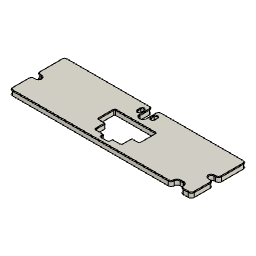
Frame Cover Plate (Autodesk Fusion 360 design; units mm, degrees)
Autodesk Fusion 360 part; units mm, degrees
sketch "Sketch1" plane through (0, 0, 0) normal (0, 0, 1) x (1, 0, 0) in component "Cover"
  line L0 (69.75, 5.3) -> (63.75, 5.3)
  line L1 (47.25, 23.3) -> (47.25, 12.3)
  line L2 (69.75, 12.3) -> (69.75, 5.3)
  line L3 (74.75, 12.3) -> (69.75, 12.3)
  line L4 (63.75, 5.3) -> (63.75, 2.8)
  line L5 (52.25, 12.3) -> (52.25, 5.3)
  line L6 (63.75, 2.8) -> (58.25, 2.8)
  line L7 (47.25, 23.3) -> (74.75, 23.3)
  line L8 (47.25, 12.3) -> (52.25, 12.3)
  line L9 (58.25, 2.8) -> (58.25, 5.3)
  line L10 (74.75, 23.3) -> (74.75, 12.3)
  line L11 (52.25, 5.3) -> (58.25, 5.3)
  circle A0 centre (12.7254, 3.937) radius 0.45 construction
  line L12 (11.8504, 5.602) -> (11.8504, 7.352) construction
  line L13 (13.6004, 5.602) -> (11.8504, 5.602) construction
  line L14 (27.5938, 3.7375) -> (27.5938, 5.5875) construction
  line L15 (29.4438, 3.7375) -> (27.5938, 3.7375) construction
  circle A1 centre (28.5188, 4.6625) radius 0.5 construction
  circle A2 centre (26.0188, 4.6625) radius 0.925 construction
  circle A3 centre (12.7254, 6.477) radius 0.45 construction
  circle A4 centre (72.7364, 31.0857) radius 1.225 construction
  circle A5 centre (77.7364, 31.0857) radius 1.225 construction
  circle A6 centre (10.1854, 6.477) radius 0.875 construction
  circle A7 centre (10.1854, 3.937) radius 0.875 construction
  circle A8 centre (43.897, 31.0857) radius 1.225 construction
  circle A9 centre (48.897, 31.0857) radius 0.7 construction
  circle A10 centre (10.1854, 3.937) radius 0.45 construction
  circle A11 centre (48.897, 31.0857) radius 1.225 construction
  circle A12 centre (10.1854, 6.477) radius 0.45 construction
  circle A13 centre (77.7364, 31.0857) radius 0.7 construction
  line L16 (11.8504, 7.352) -> (13.6004, 7.352) construction
  circle A14 centre (35.3679, 34.0015) radius 0.875 construction
  circle A15 centre (8.4979, 19.224) radius 0.925 construction
  line L17 (13.6004, 7.352) -> (13.6004, 5.602) construction
  line L18 (7.5729, 15.149) -> (9.4229, 15.149) construction
  line L19 (37.0329, 34.8765) -> (38.7829, 34.8765) construction
  line L20 (9.4229, 15.149) -> (9.4229, 13.299) construction
  line L21 (9.4229, 13.299) -> (7.5729, 13.299) construction
  circle A16 centre (35.3679, 31.4615) radius 0.45 construction
  line L22 (28.3943, 33.0249) -> (26.6443, 33.0249) construction
  circle A17 centre (37.9079, 34.0015) radius 0.45 construction
  line L23 (7.5729, 13.299) -> (7.5729, 15.149) construction
  circle A18 centre (8.4979, 16.724) radius 0.925 construction
  circle A19 centre (43.897, 31.0857) radius 0.7 construction
  circle A20 centre (23.5188, 4.6625) radius 0.5 construction
  circle A21 centre (12.7254, 3.937) radius 0.875 construction
  circle A22 centre (8.4979, 14.224) radius 0.5 construction
  circle A23 centre (72.7364, 31.0857) radius 0.7 construction
  circle A24 centre (23.5188, 4.6625) radius 0.925 construction
  line L24 (38.7829, 34.8765) -> (38.7829, 33.1265) construction
  circle A25 centre (35.3679, 34.0015) radius 0.45 construction
  line L25 (29.4438, 5.5875) -> (29.4438, 3.7375) construction
  circle A26 centre (26.0188, 4.6625) radius 0.5 construction
  line L26 (37.0329, 33.1265) -> (37.0329, 34.8765) construction
  circle A27 centre (27.5193, 31.3599) radius 0.45 construction
  line L27 (38.7829, 33.1265) -> (37.0329, 33.1265) construction
  circle A28 centre (8.4979, 19.224) radius 0.5 construction
  circle A29 centre (35.3679, 31.4615) radius 0.875 construction
  circle A30 centre (24.9793, 33.8999) radius 0.875 construction
  circle A31 centre (8.4979, 21.724) radius 0.925 construction
  line L28 (27.5938, 5.5875) -> (29.4438, 5.5875) construction
  arc A32 (83.6167, 10.5889) -> (84.2667, 10.5889) centre (83.9417, 10.5889) ccw construction
  arc A33 (83.3167, 10.6139) -> (84.5667, 10.6139) centre (83.9417, 10.6139) ccw construction
  arc A34 (79.9067, 6.3739) -> (78.6567, 6.3739) centre (79.2817, 6.3739) ccw construction
  circle A35 centre (8.4979, 16.724) radius 0.5 construction
  line L29 (26.6443, 33.0249) -> (26.6443, 34.7749) construction
  circle A36 centre (112.7141, 21.9272) radius 0.925 construction
  circle A37 centre (24.9793, 31.3599) radius 0.875 construction
  line L30 (113.6391, 13.5022) -> (111.7891, 13.5022) construction
  circle A38 centre (81.6116, 12.4939) radius 0.35 construction
  line L31 (78.6567, 6.3739) -> (78.6567, 5.8739) construction
  line L32 (43.1948, 5.6637) -> (45.0448, 5.6637) construction
  circle A39 centre (37.9079, 31.4615) radius 0.45 construction
  circle A40 centre (36.6198, 4.7387) radius 0.925 construction
  circle A41 centre (27.5193, 31.3599) radius 0.875 construction
  circle A42 centre (39.1198, 4.7387) radius 0.925 construction
  line L33 (26.6443, 34.7749) -> (28.3943, 34.7749) construction
  line L34 (28.3943, 34.7749) -> (28.3943, 33.0249) construction
  line L35 (45.0448, 3.8137) -> (43.1948, 3.8137) construction
  circle A43 centre (36.6198, 4.7387) radius 0.5 construction
  line L36 (111.7891, 15.3522) -> (113.6391, 15.3522) construction
  circle A44 centre (27.5193, 33.8999) radius 0.45 construction
  line L37 (111.7891, 13.5022) -> (111.7891, 15.3522) construction
  circle A45 centre (24.9793, 33.8999) radius 0.45 construction
  arc A46 (78.6567, 5.8739) -> (79.9067, 5.8739) centre (79.2817, 5.8739) ccw construction
  circle A47 centre (112.7141, 16.9272) radius 0.5 construction
  arc A48 (78.9567, 5.8489) -> (79.6067, 5.8489) centre (79.2817, 5.8489) ccw construction
  circle A49 centre (112.7141, 14.4272) radius 0.5 construction
  circle A50 centre (81.6116, 4.4939) radius 0.35 construction
  circle A51 centre (112.7141, 21.9272) radius 0.5 construction
  circle A52 centre (24.9793, 31.3599) radius 0.45 construction
  line L38 (113.6391, 15.3522) -> (113.6391, 13.5022) construction
  line L39 (79.9067, 5.8739) -> (79.9067, 6.3739) construction
  circle A53 centre (112.7141, 16.9272) radius 0.925 construction
  circle A54 centre (112.7141, 19.4272) radius 0.925 construction
  circle A55 centre (112.7141, 19.4272) radius 0.5 construction
  circle A56 centre (81.6116, 4.4939) radius 0.475 construction
  circle A57 centre (39.1198, 4.7387) radius 0.5 construction
  circle A58 centre (44.1198, 4.7387) radius 0.5 construction
  circle A59 centre (8.4979, 21.724) radius 0.5 construction
  line L40 (43.1948, 3.8137) -> (43.1948, 5.6637) construction
  line L41 (45.0448, 5.6637) -> (45.0448, 3.8137) construction
  line L42 (79.9067, 10.6139) -> (79.9067, 11.1139) construction
  circle A60 centre (37.9079, 31.4615) radius 0.875 construction
  circle A61 centre (41.6198, 4.7387) radius 0.5 construction
  circle A62 centre (41.6198, 4.7387) radius 0.925 construction
  circle A63 centre (81.6116, 12.4939) radius 0.475 construction
  arc A64 (84.2667, 6.3989) -> (83.6167, 6.3989) centre (83.9417, 6.3989) ccw construction
  arc A65 (84.2667, 11.1389) -> (83.6167, 11.1389) centre (83.9417, 11.1389) ccw construction
  line L43 (84.2667, 10.5889) -> (84.2667, 11.1389) construction
  arc A66 (78.9567, 10.5889) -> (79.6067, 10.5889) centre (79.2817, 10.5889) ccw construction
  line L44 (78.6567, 11.1139) -> (78.6567, 10.6139) construction
  line L45 (84.5667, 5.8739) -> (84.5667, 6.3739) construction
  line L46 (79.6067, 5.8489) -> (79.6067, 6.3989) construction
  line L47 (83.3167, 6.3739) -> (83.3167, 5.8739) construction
  arc A67 (84.5667, 11.1139) -> (83.3167, 11.1139) centre (83.9417, 11.1139) ccw construction
  arc A68 (78.6567, 10.6139) -> (79.9067, 10.6139) centre (79.2817, 10.6139) ccw construction
  arc A69 (79.6067, 6.3989) -> (78.9567, 6.3989) centre (79.2817, 6.3989) ccw construction
  arc A70 (79.9067, 11.1139) -> (78.6567, 11.1139) centre (79.2817, 11.1139) ccw construction
  line L48 (78.9567, 11.1389) -> (78.9567, 10.5889) construction
  line L49 (83.3167, 11.1139) -> (83.3167, 10.6139) construction
  arc A71 (84.5667, 6.3739) -> (83.3167, 6.3739) centre (83.9417, 6.3739) ccw construction
  line L50 (78.9567, 6.3989) -> (78.9567, 5.8489) construction
  line L51 (79.6067, 10.5889) -> (79.6067, 11.1389) construction
  line L52 (84.2667, 5.8489) -> (84.2667, 6.3989) construction
  line L53 (83.6167, 6.3989) -> (83.6167, 5.8489) construction
  line L54 (83.6167, 11.1389) -> (83.6167, 10.5889) construction
  arc A72 (79.6067, 11.1389) -> (78.9567, 11.1389) centre (79.2817, 11.1389) ccw construction
  arc A73 (83.6167, 5.8489) -> (84.2667, 5.8489) centre (83.9417, 5.8489) ccw construction
  arc A74 (83.3167, 5.8739) -> (84.5667, 5.8739) centre (83.9417, 5.8739) ccw construction
  line L55 (84.5667, 10.6139) -> (84.5667, 11.1139) construction
  line L56 (61, 23.3) -> (61, 2.8) construction
  line L57 (0, 37) -> (122, 37)
  line L58 (122, 37) -> (122, 0)
  line L59 (122, 0) -> (0, 0)
  line L60 (0, 0) -> (0, 37)
  line L61 (61, 37) -> (61, 28.5) construction
  circle A75 centre (61, 28.5) radius 2
  line L62 (63, 28.5) -> (63, 37)
  line L63 (59, 28.5) -> (59, 37)
  circle A76 centre (3, 16.5) radius 1.75
  line L64 (3, 18.25) -> (0, 18.25)
  line L65 (3, 14.75) -> (0, 14.75)
  line L66 (119, 14.75) -> (122, 14.75)
  circle A77 centre (119, 16.5) radius 1.75
  line L67 (119, 18.25) -> (122, 18.25)
  line L68 (108.5, 0) -> (108.5, 4)
  line L69 (108.5, 4) -> (114.5, 4)
  line L70 (114.5, 4) -> (114.5, 0)
  line L71 (64.5, 32.55) -> (66.5, 32.55) construction
  line L72 (66.5, 32.55) -> (66.5, 30.55)
  line L73 (66.5, 30.55) -> (64.5, 30.55) construction
  line L74 (64.5, 30.55) -> (64.5, 32.55)
  circle A78 centre (65.5, 32.55) radius 1
  circle A79 centre (65.5, 30.55) radius 1
  circle A80 centre (56.5, 32.55) radius 1
  line L75 (57.5, 30.55) -> (57.5, 32.55)
  line L76 (55.5, 32.55) -> (55.5, 30.55)
  circle A81 centre (56.5, 30.55) radius 1
  line L77 (61, 28.5) -> (61, 23.3) construction
  point P0 (111.5, 4)
  dimension "d6" = 5.5
  dimension "d8" = 7
  dimension "d9" = 2.5
  dimension "d10" = 11
  dimension "d11" = 17.5
  dimension "d14" = 122
  dimension "d15" = 37
  dimension "d16" = 8.5
  dimension "d17" = 4
  dimension "d18" = 16.5
  dimension "d19" = 3
  dimension "d20" = 3.5
  dimension "d21" = 10.5
  dimension "d22" = 4
  dimension "d23" = 6
  dimension "d24" = 2
  dimension "d26" = 4.45
  dimension "d27" = 1.5
  dimension "d29" = 2
  dimension "d39" = 27.5
  dimension "d40" = 13.7
  constraint midpoint L7 L56.start
  constraint midpoint L6 L56.end
  constraint perpendicular L7 L56
  constraint equal L0 L11
  constraint perpendicular L3 L10
  constraint perpendicular L1 L8
  constraint perpendicular L5 L8
  constraint perpendicular L0 L2
  constraint perpendicular L5 L11
  constraint perpendicular L9 L11
  constraint perpendicular L0 L4
  constraint horizontal L6
  constraint equal L3 L8
  constraint equal L1 L10
  constraint horizontal L57
  constraint vertical L58
  constraint horizontal L59
  constraint vertical L60
  constraint coincident L59.end L60.start
  constraint midpoint L57 L61.start
  constraint perpendicular L57 L61
  constraint coincident L61.end A75.centre
  constraint coincident A75 L62.start
  constraint coincident L57 L62.end
  constraint perpendicular L57 L62
  constraint coincident A75 L63.start
  constraint coincident L57 L63.end
  constraint perpendicular L57 L63
  constraint tangent A75 L62
  constraint tangent A75 L63
  constraint coincident A76 L64.start
  constraint coincident L60 L64.end
  constraint perpendicular L60 L64
  constraint coincident A76 L65.start
  constraint coincident L60 L65.end
  constraint perpendicular L60 L65
  constraint tangent A76 L65
  constraint tangent A76 L64
  constraint symmetric L61 A76 A77
  constraint symmetric L61 L64.start L67.start
  constraint symmetric L61 L64.end L67.end
  constraint symmetric L61 L65.start L66.start
  constraint symmetric L61 L65.end L66.end
  constraint coincident L59 L68.start
  constraint perpendicular L59 L68
  constraint perpendicular L68 L69
  constraint coincident L59 L70.end
  constraint perpendicular L59 L70
  constraint midpoint L69 P0
  constraint horizontal L71
  constraint vertical L72
  constraint horizontal L73
  constraint vertical L74
  constraint midpoint L71 A78.centre
  constraint coincident L71.start A78
  constraint midpoint L73 A79.centre
  constraint coincident L73.end A79
  constraint symmetric L61 L71.start L75.end
  constraint symmetric L61 L71.end L76.start
  constraint symmetric L61 L72.end L76.end
  constraint symmetric L61 L73.end L75.start
  constraint symmetric L61 A78 A80
  constraint symmetric L61 A79 A81
  constraint perpendicular L1 L7
  constraint perpendicular L7 L10
  constraint equal L2 L5
  constraint parallel L61 L77
  measures "d6" distance of L4.end L6.end
  measures "d8" distance of L0.start L2.start
  measures "d9" distance of L0.end L4.end
  measures "d10" distance of L3.start L7.end
  measures "d11" distance of L2 L5
  measures "d14" distance of L57.start L57.end
  measures "d15" distance of L57.start L59.end
  measures "d16" distance of L61.start L61.end
  measures "d17" diameter of A75
  measures "d18" distance of L59 A76.centre
  measures "d19" distance of L60 A76.centre
  measures "d20" diameter of A76
  measures "d21" distance of L58 P0
  measures "d22" distance of L69.end L70.end
  measures "d23" distance of L68.end L69.end
  measures "d24" distance of L72.end L73.end
  measures "d26" distance of L57 L71.start
  measures "d27" distance of L62 L74
  measures "d29" distance of L71.end L72.end
  measures "d39" distance of L1.start L7.end
  measures "d40" distance of L7 L57
extrude "Extrude1" add sketch "Sketch1" against normal blind 3.2 contours L57 L58 L59 L60 A75 L62 L63 A76 L64 L65 L66 A77 L67 L68 L69 L70 in component "Cover"
sketch "Sketch2" plane through (0, 0, 0) normal (0, 0, 1) x (1, 0, 0) in component "Cover"
  line L0 (6.4449, 24.826) -> (10.7371, 24.826)
  line L1 (10.7371, 24.826) -> (10.7371, 11.234)
  line L2 (10.7371, 11.234) -> (6.4449, 11.234)
  line L3 (6.4449, 11.234) -> (6.4449, 24.826)
  line L4 (22.8984, 35.6588) -> (52.6326, 35.6588)
  line L5 (52.6326, 35.6588) -> (52.6326, 28.8117)
  line L6 (52.6326, 28.8117) -> (22.8984, 28.8117)
  line L7 (22.8984, 28.8117) -> (22.8984, 35.6588)
  line L8 (69.5854, 33.9215) -> (80.3325, 33.9215)
  line L9 (80.3325, 33.9215) -> (80.3325, 27.119)
  line L10 (80.3325, 27.119) -> (69.5854, 27.119)
  line L11 (69.5854, 27.119) -> (69.5854, 33.9215)
  line L12 (109.8642, 24.5376) -> (115.4271, 24.5376)
  line L13 (115.4271, 24.5376) -> (115.4271, 11.234)
  line L14 (115.4271, 11.234) -> (109.8642, 11.234)
  line L15 (109.8642, 11.234) -> (109.8642, 24.5376)
  line L16 (77.5776, 14.2844) -> (86.1946, 14.2844)
  line L17 (86.1946, 14.2844) -> (86.1946, 2.5042)
  line L18 (86.1946, 2.5042) -> (77.5776, 2.5042)
  line L19 (77.5776, 2.5042) -> (77.5776, 14.2844)
  line L20 (8.2048, 8.3943) -> (46.1635, 8.3943)
  line L21 (46.1635, 8.3943) -> (46.1635, 2.5042)
  line L22 (46.1635, 2.5042) -> (8.2048, 2.5042)
  line L23 (8.2048, 2.5042) -> (8.2048, 8.3943)
  line L24 (47.5119, 12.3264) -> (47.5119, 23.3264)
  line L25 (47.5119, 23.3264) -> (75.0119, 23.3264)
  line L26 (75.0119, 23.3264) -> (75.0119, 12.3264)
  line L27 (75.0119, 12.3264) -> (69.7619, 12.3264)
  line L28 (69.7619, 12.3264) -> (69.7619, 5.3264)
  line L29 (69.7619, 5.3264) -> (64.0119, 5.3264)
  line L30 (64.0119, 5.3264) -> (64.0119, 2.8264)
  line L31 (64.0119, 2.8264) -> (58.5119, 2.8264)
  line L32 (58.5119, 2.8264) -> (58.5119, 5.3264)
  line L33 (58.5119, 5.3264) -> (52.7619, 5.3264)
  line L34 (52.7619, 5.3264) -> (52.7619, 12.3264)
  line L35 (52.7619, 12.3264) -> (47.5119, 12.3264)
  arc A0 (64.5, 30.55) -> (66.5, 30.55) centre (65.5, 30.55) ccw
  line L36 (64.5, 30.55) -> (64.5, 32.55)
  arc A1 (66.5, 32.55) -> (64.5, 32.55) centre (65.5, 32.55) ccw
  line L37 (66.5, 32.55) -> (66.5, 30.55)
  arc A2 (57.5, 32.55) -> (55.5, 32.55) centre (56.5, 32.55) ccw
  line L38 (57.5, 32.55) -> (57.5, 30.55)
  arc A3 (55.5, 30.55) -> (57.5, 30.55) centre (56.5, 30.55) ccw
  line L39 (55.5, 30.55) -> (55.5, 32.55)
  line L40 (108.5, 0) -> (108.5, 4)
  line L41 (108.5, 4) -> (114.5, 4)
  line L42 (114.5, 4) -> (114.5, 0)
  line L43 (114.5, 0) -> (122, 0)
  line L44 (122, 0) -> (122, 14.75)
  line L45 (122, 14.75) -> (119, 14.75)
  arc A4 (119, 18.25) -> (119, 14.75) centre (119, 16.5) ccw
  line L46 (119, 18.25) -> (122, 18.25)
  line L47 (122, 18.25) -> (122, 37)
  line L48 (122, 37) -> (63, 37)
  line L49 (63, 37) -> (63, 28.5)
  arc A5 (59, 28.5) -> (63, 28.5) centre (61, 28.5) ccw
  line L50 (59, 28.5) -> (59, 37)
  line L51 (59, 37) -> (0, 37)
  line L52 (0, 37) -> (0, 18.25)
  line L53 (0, 18.25) -> (3, 18.25)
  arc A6 (3, 14.75) -> (3, 18.25) centre (3, 16.5) ccw
  line L54 (3, 14.75) -> (0, 14.75)
  line L55 (0, 14.75) -> (0, 0)
  line L56 (0, 0) -> (108.5, 0)
  arc A7 (64.5, 30.55) -> (66.5, 30.55) centre (65.5, 30.55) ccw
  line L57 (64.5, 30.55) -> (64.5, 32.55)
  arc A8 (66.5, 32.55) -> (64.5, 32.55) centre (65.5, 32.55) ccw
  line L58 (66.5, 32.55) -> (66.5, 30.55)
  line L59 (47.25, 12.3) -> (47.25, 23.3)
  line L60 (47.25, 23.3) -> (74.75, 23.3)
  line L61 (74.75, 23.3) -> (74.75, 12.3)
  line L62 (74.75, 12.3) -> (69.75, 12.3)
  line L63 (69.75, 12.3) -> (69.75, 5.3)
  line L64 (69.75, 5.3) -> (63.75, 5.3)
  line L65 (63.75, 5.3) -> (63.75, 2.8)
  line L66 (63.75, 2.8) -> (58.25, 2.8)
  line L67 (58.25, 2.8) -> (58.25, 5.3)
  line L68 (58.25, 5.3) -> (52.25, 5.3)
  line L69 (52.25, 5.3) -> (52.25, 12.3)
  line L70 (52.25, 12.3) -> (47.25, 12.3)
  arc A9 (57.5, 32.55) -> (55.5, 32.55) centre (56.5, 32.55) ccw
  line L71 (57.5, 32.55) -> (57.5, 30.55)
  arc A10 (55.5, 30.55) -> (57.5, 30.55) centre (56.5, 30.55) ccw
  line L72 (55.5, 30.55) -> (55.5, 32.55)
  line L73 (108.5, 0) -> (108.5, 4)
  line L74 (108.5, 4) -> (114.5, 4)
  line L75 (114.5, 4) -> (114.5, 0)
  line L76 (114.5, 0) -> (122, 0)
  line L77 (122, 0) -> (122, 14.75)
  line L78 (122, 14.75) -> (119, 14.75)
  arc A11 (119, 18.25) -> (119, 14.75) centre (119, 16.5) ccw
  line L79 (119, 18.25) -> (122, 18.25)
  line L80 (122, 18.25) -> (122, 37)
  line L81 (122, 37) -> (63, 37)
  line L82 (63, 37) -> (63, 28.5)
  arc A12 (59, 28.5) -> (63, 28.5) centre (61, 28.5) ccw
  line L83 (59, 28.5) -> (59, 37)
  line L84 (59, 37) -> (0, 37)
  line L85 (0, 37) -> (0, 18.25)
  line L86 (0, 18.25) -> (3, 18.25)
  arc A13 (3, 14.75) -> (3, 18.25) centre (3, 16.5) ccw
  line L87 (3, 14.75) -> (0, 14.75)
  line L88 (0, 14.75) -> (0, 0)
  line L89 (0, 0) -> (108.5, 0)
  line L90 (70.3619, 1) -> (73.1619, 1)
  line L91 (73.1619, 1) -> (73.1619, 6)
  line L92 (73.1619, 6) -> (70.3619, 6)
  line L93 (70.3619, 6) -> (70.3619, 1)
  line L94 (61.2619, 2.8264) -> (61.2619, 0) construction
  line L95 (71.7619, 1) -> (71.7619, 0) construction
  dimension "d33" = 10.5
  dimension "d34" = 5
  dimension "d35" = 2.8
  dimension "d36" = 1
  constraint horizontal L0
  constraint vertical L1
  constraint horizontal L2
  constraint vertical L3
  constraint horizontal L4
  constraint vertical L5
  constraint horizontal L6
  constraint vertical L7
  constraint horizontal L8
  constraint vertical L9
  constraint horizontal L10
  constraint vertical L11
  constraint horizontal L12
  constraint vertical L13
  constraint horizontal L14
  constraint vertical L15
  constraint horizontal L16
  constraint vertical L17
  constraint horizontal L18
  constraint vertical L19
  constraint horizontal L20
  constraint vertical L21
  constraint horizontal L22
  constraint vertical L23
  constraint horizontal L90
  constraint vertical L91
  constraint horizontal L92
  constraint vertical L93
  constraint midpoint L31 L94.start
  constraint coincident L89 L94.end
  constraint perpendicular L89 L94
  constraint midpoint L90 L95.start
  constraint coincident L56 L95.end
  constraint perpendicular L56 L95
  measures "d33" distance of L94.end L95.end
  measures "d34" distance of L90.end L91.end
  measures "d35" distance of L91.end L92.end
  measures "d36" distance of L56 L90
extrude "Extrude2" cut sketch "Sketch2" along normal blind 2 from surface at -3.2 contours L0 L1 L2 L3 | L4 L5 L6 L7 | L8 L9 L10 L11 | L12 L13 L14 L15 | L20 L21 L22 L23 | L90 L91 L92 L93 in component "Cover"
fillet "Fillet1" radius 2 14 edges at (59, 37, -1.6) (63, 37, -1.6) (0, 18.25, -1.6) (0, 14.75, -1.6) (0, 37, -1.6) (0, 0, -1.6) (122, 37, -1.6) (122, 18.25, -1.6) (122, 14.75, -1.6) (122, 0, -1.6) (114.5, 0, -1.6) (108.5, 0, -1.6) (108.5, 4, -1.6) (114.5, 4, -1.6) in component "Cover"
fillet "Fillet2" radius 0.6 16 edges at (52.25, 5.3, -1.6) (58.25, 2.8, -1.6) (63.75, 2.8, -1.6) (69.75, 5.3, -1.6) (74.75, 12.3, -1.6) (47.25, 12.3, -1.6) (47.25, 23.3, -1.6) (74.75, 23.3, -1.6) (52.25, 12.3, -1.6) (69.75, 12.3, -1.6) (58.25, 5.3, -1.6) (63.75, 5.3, -1.6) (70.3619, 6, -2.2) (70.3619, 1, -2.2) (73.1619, 1, -2.2) (73.1619, 6, -2.2) in component "Cover"
chamfer "Chamfer1" distance 0.4 angle 45 1 faces at (104.0631, 25.7682, 0) in component "Cover"
component "Cover" placed x (1, 0, 0) y (0, 1, 0) z (0, 0, 1) at (0, 0, 0)
